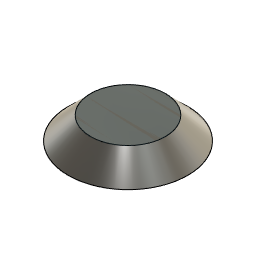
Top cover (Autodesk Fusion 360 design; units mm, degrees)
Autodesk Fusion 360 part; units mm, degrees
sketch "Sketch1" plane through (0, 0, 0) normal (1, 0, 0) x (0, 1, 0)
  line L0 (0, 76.107) -> (0, -44.382) construction
  line L1 (0, 0) -> (0, 30)
  line L2 (0, 30) -> (50, 30)
  line L3 (0, 0) -> (80, 0)
  line L4 (50, 30) -> (80, 0)
  dimension "d1" = 30
  dimension "d2" = 50
  dimension "d3" = 80
  constraint vertical L0
  constraint coincident L1.start L3.start
  constraint parallel L0 L1
  constraint perpendicular L1 L2
  constraint perpendicular L1 L3
  measures "d1" distance of L1.start L1.end
  measures "d2" distance of L1.end L2.end
  measures "d3" distance of L1.start L3.end
revolve "Revolve1" add sketch "Sketch1" angle 360 about axis through (0, 0, 76.107) along (0, 0, -1)
shell "Shell1" thickness 1.2 removed faces 1 at (-12.9887, 15.4417, 0)
sketch "Sketch3" plane through (0, 0, 28.8) normal (0, 0, -1) x (1, 0, 0)
  circle A0 centre (0, 0) radius 49.5029
  circle A1 centre (0, 0) radius 30 construction
  line L0 (0, 0) -> (-25.6418, 25.6418) construction
  line L1 (0, 0) -> (36.263, 0) construction
  circle A2 centre (-21.2132, 21.2132) radius 4
  circle A3 centre (-21.2132, 21.2132) radius 2
  circle A4 centre (-21.2132, -21.2132) radius 4
  circle A5 centre (-21.2132, -21.2132) radius 2
  circle A6 centre (21.2132, -21.2132) radius 4
  circle A7 centre (21.2132, -21.2132) radius 2
  circle A8 centre (21.2132, 21.2132) radius 4
  circle A9 centre (21.2132, 21.2132) radius 2
  circle A10 centre (0, 0) radius 2
  dimension "d26" = 60
  dimension "d27" = 135
  dimension "d28" = 8
  dimension "d29" = 4
  dimension "d31" = 360
  dimension "d32" = 4
  constraint coincident A0.centre A1.centre
  constraint horizontal L1
  constraint coincident L0 A2.centre
  constraint coincident A1 A2.centre
  constraint concentric A2 A3
  measures "d26" diameter of A1
  measures "d27" angle of L0 L1
  measures "d28" diameter of A2
  measures "d29" diameter of A3
  measures "d32" diameter of A10
extrude "Extrude4" add sketch "Sketch3" along normal blind 15 contours A2 | A6
extrude "Extrude5" add sketch "Sketch3" along normal blind 10 contours A4 | A8
sketch "Sketch4" plane through (0, 0, 30) normal (0, 0, 1) x (-1, 0, 0)
  circle A0 centre (0, 0) radius 50
